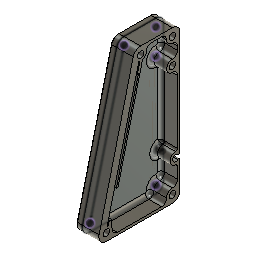
enclosure (Autodesk Fusion 360 design; units mm, degrees)
Autodesk Fusion 360 part; units mm, degrees
sketch "base-measurements" plane through (0, 0, 0) normal (1, 0, 0) x (0, 1, 0)
  circle A0 centre (0, 0) radius 2.55
  circle A1 centre (0, 108) radius 2.55
  circle A2 centre (-25.072576, 108) radius 2.55
  circle A3 centre (-52, 0) radius 2.55
  line L0 (0, 108) -> (-25.072576, 108) construction
  line L1 (-25.072576, 108) -> (-52, 0) construction
  line L2 (-52, 0) -> (0, 0) construction
  circle A4 centre (0, 88) radius 2.55
  line L3 (0, 0) -> (0, 88) construction
  line L4 (0, 88) -> (0, 108) construction
  dimension "rodOuterDiameter" = 5.1
  dimension "d2" = 5.1
  dimension "d3" = 5.1
  dimension "d4" = 5.1
  dimension "d8" = 52
  dimension "d9" = 108
  dimension "d105" = 76
  dimension "d108" = 5.1
  dimension "d134" = 20
  constraint coincident A0.centre L2.end
  constraint coincident A1.centre L0.start
  constraint horizontal L0
  constraint coincident A3.centre L1.end
  constraint horizontal L2
  constraint coincident A4.centre L3.end
  constraint vertical L4
  constraint vertical L3
  measures "rodOuterDiameter" diameter of A0
  measures "d2" diameter of A1
  measures "d3" diameter of A2
  measures "d4" diameter of A3
  measures "d8" distance of A0.centre A3.centre
  measures "d9" distance of A0.centre A1.centre
  measures "d105" angle of L1 L2
  measures "d108" diameter of A4
  measures "d134" distance of A1.centre A4.centre
sketch "left-panel-outline" plane through (0, 0, 0) normal (1, 0, 0) x (0, 1, 0)
  line L0 (-52, -6) -> (0, -6)
  line L1 (0, 114) -> (-25.072576, 114)
  line L2 (-30.89435, 109.451531) -> (-57.821774, 1.451531)
  arc A0 (0, -6) -> (6, 0) centre (0, 0) ccw
  arc A1 (-57.821774, 1.451531) -> (-52, -6) centre (-52, 0) ccw
  arc A2 (6, 108) -> (0, 114) centre (0, 108) ccw
  arc A3 (-25.072576, 114) -> (-30.89435, 109.451531) centre (-25.072576, 108) ccw
  circle A4 centre (0, 108) radius 2.55
  circle A5 centre (-25.072576, 108) radius 2.55
  circle A6 centre (0, 0) radius 2.55
  circle A7 centre (-52, 0) radius 2.55
  circle A8 centre (-25.072576, 108) radius 1.75
  circle A9 centre (0, 108) radius 1.75
  circle A10 centre (0, 0) radius 1.75
  circle A11 centre (-52, 0) radius 1.75
  line L3 (-26.513946, 104.079095) -> (-51.431901, 4.138636)
  line L4 (-26.513946, 104.079095) -> (-25.64068, 103.861366)
  line L5 (-25.640679, 103.861365) -> (-50.558634, 3.920906)
  line L6 (-50.558634, 3.920906) -> (-51.4319, 4.138635)
  line L7 (-25.072578, 108.000001) -> (-26.077313, 103.970231) construction
  line L8 (-52.000001, 0) -> (-50.995267, 4.02977) construction
  circle A12 centre (0, 88) radius 1.75
  circle A13 centre (0, 88) radius 2.55
  line L9 (6, 0) -> (6, 21)
  line L10 (6, 108) -> (6, 26.25)
  arc A14 (4.338562, 25.5) -> (6, 26.25) centre (5, 26.25) ccw
  arc A15 (6, 21) -> (4.338562, 21.75) centre (5, 21) ccw
  arc A16 (4.338562, 25.5) -> (4.338562, 21.75) centre (2.684968, 23.625) ccw
  line L11 (5, 26.25) -> (5, 21) construction
  dimension "d10" = 6
  dimension "screwHole" = 3.5
  dimension "d12" = 3.5
  dimension "d13" = 3.5
  dimension "d14" = 3.5
  dimension "d17" = 103
  dimension "d18" = 0.9
  dimension "d110" = 3.5
  dimension "d122" = 2.5
  dimension "d123" = 1
  dimension "d124" = 21
  dimension "d125" = 5.25
  constraint horizontal L0
  constraint horizontal L1
  constraint tangent L0 A0
  constraint tangent L0 A1
  constraint tangent L1 A2
  constraint tangent L1 A3
  constraint concentric A2 A4
  constraint concentric A3 A5
  constraint concentric A0 A6
  constraint concentric A1 A7
  constraint tangent L2 A1
  constraint tangent L2 A3
  constraint concentric A3 A8
  constraint concentric A4 A9
  constraint concentric A6 A10
  constraint concentric A1 A11
  constraint parallel L3 L5
  constraint perpendicular L5 L6
  constraint perpendicular L3 L4
  constraint coincident A1.centre A7.centre
  constraint equal L7 L8
  constraint parallel L2 L3
  constraint parallel L3 L8
  constraint concentric A12 A13
  constraint tangent A0 L9
  constraint vertical L9
  constraint tangent A2 L10
  constraint vertical L10
  constraint tangent L10 A14
  constraint tangent L9 A15
  constraint tangent A15 A16
  constraint tangent A14 A16
  constraint equal A14 A15
  constraint coincident A14.centre L11.start
  constraint coincident A15.centre L11.end
  constraint vertical L11
  measures "d10" radius of A2
  measures "screwHole" diameter of A8
  measures "d12" diameter of A9
  measures "d13" diameter of A10
  measures "d14" diameter of A11
  measures "d110" diameter of A12
  measures "d122" radius of A16
  measures "d123" radius of A14
  measures "d124" distance of A0.end L9.end
  measures "d125" distance of A14.centre A15.centre
extrude "Extrude1" add sketch "left-panel-outline" against normal blind 5 contours L0 L1 L2 A0 A1 A2 A3 L9 L10 A14 A15 A16 | A4 | A5 | A6 | A7 | L3 L4 L5 L6 | A13 picked at (-17.305036, 38.349698) picked at (-1.246633, 109.90586) picked at (-23.825943, 109.90586) picked at (2.267324, -0.213627) picked at (-49.732676, -0.213627) picked at (-42.543738, 37.306969) picked at (-1.246633, 89.90586) makes body 1
extrude "Extrude2" add sketch "left-panel-outline" along normal blind 13 contours L0 L1 L2 A0 A1 A2 A3 L9 L10 A14 A15 A16 picked at (-17.305036, 38.349698) bodies 1
sketch "left-panel-recess" plane through (13, 0, 0) normal (1, 0, 0) x (0, 1, 0)
  circle A0 centre (-25.072576, 108) radius 2.55
  circle A1 centre (0, 108) radius 2.55
  circle A2 centre (0, 0) radius 2.55
  circle A3 centre (-52, 0) radius 2.55
  line L0 (-51.4319, 4.138635) -> (-26.513946, 104.079095)
  line L1 (-26.513946, 104.079095) -> (-25.640679, 103.861365)
  line L2 (-25.640679, 103.861365) -> (-50.558634, 3.920906)
  line L3 (-50.558634, 3.920906) -> (-51.4319, 4.138635)
  arc A4 (-25.072576, 114) -> (-30.89435, 109.451531) centre (-25.072576, 108) ccw
  line L4 (-30.89435, 109.451531) -> (-57.821774, 1.451531)
  arc A5 (-57.821774, 1.451531) -> (-52, -6) centre (-52, 0) ccw
  line L5 (-52, -6) -> (0, -6)
  arc A6 (0, -6) -> (6, 0) centre (0, 0) ccw
  arc A7 (6, 108) -> (0, 114) centre (0, 108) ccw
  line L6 (0, 114) -> (-25.072576, 114)
  line L7 (-23.747087, 103.189014) -> (-42.942712, 26.199571)
  line L8 (-43.45, -4) -> (-8.55, -4)
  arc A8 (0, 4.55) -> (-4.55, 0) centre (0, 0) ccw
  arc A9 (0, 4.55) -> (4, 8.55) centre (0, 8.55) ccw
  arc A10 (-8.55, -4) -> (-4.55, 0) centre (-8.55, 0) ccw
  arc A11 (-4.55, 108) -> (0, 103.45) centre (0, 108) ccw
  arc A12 (4, 99.45) -> (0, 103.45) centre (0, 99.45) ccw
  line L9 (-16.522576, 112) -> (-8.55, 112)
  arc A13 (-4.55, 108) -> (-8.55, 112) centre (-8.55, 108) ccw
  line L10 (-50.558634, 3.920906) -> (-25.640679, 103.861365)
  arc A14 (-23.190446, 103.857526) -> (-20.522576, 108) centre (-25.072576, 108) ccw
  arc A15 (-16.522576, 112) -> (-20.522576, 108) centre (-16.522576, 108) ccw
  arc A16 (-23.190446, 103.857526) -> (-23.747087, 103.189014) centre (-22.77679, 102.947091) ccw
  arc A17 (-47.45, 0) -> (-47.94694, 2.067657) centre (-52, 0) ccw
  arc A18 (-47.45, 0) -> (-43.45, -4) centre (-43.45, 0) ccw
  line L11 (-48.264993, 4.853065) -> (-47.781149, 6.793656)
  arc A19 (-48.264993, 4.853065) -> (-47.94694, 2.067657) centre (-44.38381, 3.885377) ccw
  line L12 (-44.155581, 26.501973) -> (-26.848332, 95.917558)
  line L13 (-26.848332, 95.917558) -> (-27.576054, 96.099)
  line L14 (-42.942712, 26.199571) -> (-44.155581, 26.501973)
  line L15 (-47.781149, 6.793656) -> (-49.721741, 7.2775)
  line L16 (4, 99.45) -> (4, 96.55)
  arc A20 (4, 79.45) -> (0, 83.45) centre (0, 79.45) ccw
  arc A21 (0, 92.55) -> (4, 96.55) centre (0, 96.55) ccw
  arc A22 (0, 92.55) -> (0, 83.45) centre (0, 88) ccw
  circle A23 centre (0, 88) radius 2.55
  circle A24 centre (0, 88) radius 2.55
  line L17 (6, 0) -> (6, 21)
  arc A25 (6, 21) -> (4.338562, 21.75) centre (5, 21) ccw
  arc A26 (4.338562, 25.5) -> (4.338562, 21.75) centre (2.684968, 23.625) ccw
  arc A27 (4.338562, 25.5) -> (6, 26.25) centre (5, 26.25) ccw
  line L18 (6, 26.25) -> (6, 108)
  arc A28 (2.546242, 28.122861) -> (2.546242, 19.127139) centre (2.684968, 23.625) ccw
  arc A29 (2.546242, 28.122861) -> (4, 29.622148) centre (2.5, 29.622148) ccw
  arc A30 (4, 17.627852) -> (2.546242, 19.127139) centre (2.5, 17.627852) ccw
  line L19 (4, 17.627852) -> (4, 8.55)
  line L20 (4, 29.622148) -> (4, 79.45)
  dimension "d28" = 2
  dimension "d29" = 4
  dimension "d31" = 2
  dimension "d33" = 2
  dimension "d34" = 2
  dimension "d35" = 1
  dimension "d50" = 2
  dimension "d59" = 0.75
  dimension "d60" = 8
  dimension "d71" = 20
  dimension "d112" = 2
  dimension "d117" = 2
  dimension "d118" = 2
  dimension "d119" = 2
  dimension "d126" = 2
  dimension "d127" = 2
  dimension "d128" = 2
  dimension "d129" = 2
  dimension "d130" = 1.5
  constraint horizontal L8
  constraint tangent A8 A9
  constraint tangent A8 A10
  constraint tangent L8 A10
  constraint equal A9 A10
  constraint tangent A11 A12
  constraint equal A9 A12
  constraint horizontal L9
  constraint tangent L9 A13
  constraint equal A12 A13
  constraint tangent A11 A13
  constraint parallel L2 L7
  constraint concentric A0 A14
  constraint tangent A14 A15
  constraint tangent L9 A15
  constraint equal A13 A15
  constraint tangent L7 A16
  constraint tangent A14 A16
  constraint tangent L8 A18
  constraint tangent A17 A18
  constraint equal A10 A18
  constraint tangent L11 A19
  constraint collinear L7 L11
  constraint tangent A17 A19
  constraint equal A18 A19
  constraint perpendicular L2 L13
  constraint perpendicular L12 L13
  constraint perpendicular L12 L14
  constraint perpendicular L2 L15
  constraint tangent A12 L16
  constraint tangent L16 A21
  constraint concentric A22 A23
  constraint coincident A20.end A22.end
  constraint tangent A21 A22
  constraint tangent A20 A22
  constraint equal A12 A21
  constraint equal A20 A21
  constraint tangent A28 A29
  constraint tangent A28 A30
  constraint vertical L19
  constraint tangent A30 L19
  constraint vertical L20
  constraint tangent A29 L20
  constraint coincident A20.start L20.end
  constraint tangent A20 L20
  constraint equal A29 A30
  constraint tangent A9 L19
  measures "d28" distance of L5 L8
  measures "d29" radius of A9
  measures "d31" distance of L6 L9
  measures "d33" distance of L7 L10
  measures "d34" distance of A0 A14
  measures "d35" radius of A16
  measures "d71" distance of L14 L15
  measures "d112" distance of A22 A23
  measures "d117" distance of A1 A11
  measures "d118" distance of A2 A8
  measures "d119" distance of A3 A17
  measures "d126" distance of L16 L18
  measures "d127" distance of L18 L20
  measures "d128" distance of L17 L19
  measures "d129" distance of A26 A28
  measures "d130" radius of A29
extrude "Extrude3" cut sketch "left-panel-recess" against normal blind 13 contours L2 L7 L8 A8 A9 A10 A11 A12 L9 A13 L10 A14 A15 A16 A17 A18 L11 A19 L12 L13 L14 L15 L16 A20 A21 A22 A28 A29 A30 L19 L20 picked at (-15.142097, 45.9114) bodies 1
ref_plane "WorkPlane1" through (151, -23.715951, 54) normal (1, 0, 0) x (0, 1, 0)
sketch "right-panel" plane through (151, 0, 0) normal (1, 0, 0) x (0, 1, 0)
  arc A0 (6, 108) -> (0, 114) centre (0, 108) ccw
  line L0 (0, 114) -> (-25.072576, 114)
  arc A1 (-25.072576, 114) -> (-30.89435, 109.451531) centre (-25.072576, 108) ccw
  line L1 (-30.89435, 109.451531) -> (-57.821774, 1.451531)
  arc A2 (-57.821774, 1.451531) -> (-52, -6) centre (-52, 0) ccw
  line L2 (-52, -6) -> (0, -6)
  arc A3 (0, -6) -> (6, 0) centre (0, 0) ccw
  circle A4 centre (-25.072576, 108) radius 2.55
  circle A5 centre (-25.072576, 108) radius 1.75
  circle A6 centre (0, 108) radius 2.55
  circle A7 centre (0, 108) radius 1.75
  line L3 (-26.513946, 104.079095) -> (-51.431901, 4.138636)
  line L4 (-26.513946, 104.079095) -> (-25.64068, 103.861366)
  line L5 (-50.558634, 3.920906) -> (-51.4319, 4.138635)
  line L6 (-25.640679, 103.861365) -> (-50.558634, 3.920906)
  circle A8 centre (0, 0) radius 2.55
  circle A9 centre (0, 0) radius 1.75
  circle A10 centre (-52, 0) radius 2.55
  circle A11 centre (-52, 0) radius 1.75
  line L7 (-52, 0) -> (-50.995267, 4.02977)
  line L8 (-25.072578, 108.000001) -> (-26.077313, 103.970231)
  circle A12 centre (0, 88) radius 2.55
  circle A13 centre (0, 88) radius 1.75
  line L9 (6, 108) -> (6, 0)
  constraint coincident A0.start L9.start
  constraint coincident A3.end L9.end
extrude "Extrude6" add sketch "right-panel" along normal blind 5 separate body contours A0 L0 A1 L1 A2 L2 A3 L9 | A4 | A6 | L3 L4 L5 L6 | A8 | A10 | A12 picked at (-17.702878, 30.640302) picked at (-25.745071, 105.824135) picked at (-1.246633, 109.90586) picked at (-42.834827, 37.379546) picked at (2.267324, -0.213627) picked at (-50.655141, 1.838083) picked at (-1.246633, 89.90586) makes body 2
extrude "Extrude7" add sketch "right-panel" against normal blind 13 separate body contours A0 L0 A1 L1 A2 L2 A3 L9 picked at (-17.702878, 30.640302) makes body 3
extrude "Extrude8" add sketch "right-panel" against normal blind 9.5 contours L3 L4 L5 L6 picked at (-42.834827, 37.379546) bodies 2 3
sketch "right-panel-recess" plane through (138, 0, 0) normal (-1, 0, 0) x (0, -1, 0)
  circle A0 centre (25.072576, 108) radius 2.55
  circle A1 centre (0, 0) radius 2.55
  line L0 (26.513946, 104.079095) -> (51.4319, 4.138635)
  line L1 (51.4319, 4.138635) -> (50.558634, 3.920906)
  line L2 (50.558634, 3.920906) -> (25.640679, 103.861365)
  line L3 (25.640679, 103.861365) -> (26.513946, 104.079095)
  circle A2 centre (52, 0) radius 2.55
  circle A3 centre (0, 108) radius 2.55
  arc A4 (-6, 0) -> (0, -6) centre (0, 0) ccw
  line L4 (0, -6) -> (52, -6)
  arc A5 (52, -6) -> (57.821774, 1.451531) centre (52, 0) ccw
  line L5 (57.821774, 1.451531) -> (30.89435, 109.451531)
  arc A6 (30.89435, 109.451531) -> (25.072576, 114) centre (25.072576, 108) ccw
  line L6 (25.072576, 114) -> (0, 114)
  arc A7 (0, 114) -> (-6, 108) centre (0, 108) ccw
  arc A8 (47.94694, 2.067657) -> (47.45, 0) centre (52, 0) ccw
  arc A9 (43.45, -4) -> (47.45, 0) centre (43.45, 0) ccw
  line L7 (43.45, -4) -> (8.55, -4)
  arc A10 (4.55, 0) -> (8.55, -4) centre (8.55, 0) ccw
  arc A11 (4.55, 0) -> (0, 4.55) centre (0, 0) ccw
  arc A12 (-4, 8.55) -> (0, 4.55) centre (0, 8.55) ccw
  arc A13 (0, 103.45) -> (-4, 99.45) centre (0, 99.45) ccw
  arc A14 (0, 103.45) -> (4.55, 108) centre (0, 108) ccw
  arc A15 (8.55, 112) -> (4.55, 108) centre (8.55, 108) ccw
  line L8 (16.522576, 112) -> (8.55, 112)
  arc A16 (20.522576, 108) -> (16.522576, 112) centre (16.522576, 108) ccw
  line L9 (23.858089, 102.743812) -> (48.264993, 4.853065)
  arc A17 (20.522576, 108) -> (22.880881, 104.012648) centre (25.072576, 108) ccw
  arc A18 (23.858089, 102.743812) -> (22.880881, 104.012648) centre (21.9175, 102.259969) ccw
  arc A19 (47.94694, 2.067657) -> (48.264993, 4.853065) centre (44.38381, 3.885377) ccw
  arc A20 (0, 83.45) -> (-4, 79.45) centre (0, 79.45) ccw
  arc A21 (0, 83.45) -> (0, 92.55) centre (0, 88) ccw
  arc A22 (-4, 96.55) -> (0, 92.55) centre (0, 96.55) ccw
  line L10 (-4, 99.45) -> (-4, 96.55)
  circle A23 centre (0, 88) radius 2.55
  circle A24 centre (0, 88) radius 2.55
  line L11 (-6, 108) -> (-6, 0)
  line L12 (-4, 79.45) -> (-4, 8.55)
  point P0 (0, 88)
  dimension "d67" = 2
  dimension "d68" = 2
  constraint parallel L2 L9
  constraint concentric A0 A17
  constraint tangent A17 A18
  constraint tangent L9 A18
  constraint tangent L9 A19
  constraint tangent A8 A19
  constraint coincident A20.end L12.start
  constraint coincident A12.start L12.end
  measures "d67" distance of L2 L9
  measures "d68" radius of A18
extrude "Extrude9" cut sketch "right-panel-recess" against normal blind 13.5 contours A8 A9 L7 A10 A11 A12 A13 A14 A15 L8 A16 L9 A17 A18 A19 A20 A21 A22 L10 L12 picked at (13.421664, 30.951022) bodies 2
fillet "Fillet1" radius 3 25 edges at (0, -33.3449, 64.694292) (0, -23.545268, 103.58697) (0, -21.247253, 105.536384) (0, -19.351003, 110.828427) (0, -12.536288, 112) (0, -5.721573, 110.828427) (0, -3.217336, 104.782664) (0, 2.828427, 102.278427) (0, 4, 98) (0, 2.828427, 93.721573) (0, -4.55, 88) (0, 2.828427, 82.278427) (0, 4, 54.536074) (0, 3.576885, 28.577965) (0, -1.815032, 23.625) (0, 3.576885, 18.672035) (0, 4, 13.088926) (0, 2.828427, 5.721573) (0, -3.217336, 3.217336) (0, -5.721573, -2.828427) (0, -26, -4) (0, -46.278427, -2.828427) (0, -47.575979, 1.063268) (0, -48.357986, 3.431584) (0, -48.023071, 5.82336) on bodies 1
fillet "Fillet2" radius 3 20 edges at (151.5, -3.217336, 104.782664) (151.5, -5.721573, 110.828427) (151.5, -12.536288, 112) (151.5, -19.351003, 110.828427) (151.5, -21.156282, 105.683722) (151.5, -23.502034, 103.480314) (151.5, -36.061541, 53.798438) (151.5, -48.357986, 3.431584) (151.5, -47.575979, 1.063268) (151.5, -46.278427, -2.828427) (151.5, -26, -4) (151.5, -5.721573, -2.828427) (151.5, -3.217336, 3.217336) (151.5, 2.828427, 5.721573) (151.5, 4, 44) (151.5, 2.828427, 82.278427) (151.5, -4.55, 88) (151.5, 2.828427, 93.721573) (151.5, 4, 98) (151.5, 2.828427, 102.278427) on bodies 2
sketch "rpi-support-bar" plane through (0, 0, 0) normal (1, 0, 0) x (0, 1, 0)
  arc A0 (6, 88) -> (-1.764706, 82.265385) centre (0, 88) ccw
  line L0 (0, 79.875962) -> (0, 8.124038)
  arc A1 (0, 79.875962) -> (-1.764706, 82.265385) centre (-2.5, 79.875962) ccw
  circle A2 centre (0, 0) radius 2.55 construction
  arc A3 (-1.764706, 5.734615) -> (6, -0.000003) centre (0, 0) ccw
  arc A4 (-1.764706, 5.734615) -> (0, 8.124038) centre (-2.5, 8.124038) ccw
  line L1 (0, 0) -> (0, -6) construction
  circle A5 centre (0, 88) radius 2.55
  circle A6 centre (0, 0) radius 2.55
  circle A7 centre (0, 88) radius 2.55
  line L2 (6, -0.000003) -> (6, 88)
  arc A8 (0, -6) -> (6, 0) centre (0, 0) ccw
  dimension "d100" = 2.5
  dimension "d133" = 6
  constraint vertical L0
  constraint tangent L0 A1
  constraint coincident A2.centre A3.centre
  constraint tangent L0 A4
  constraint coincident A3 L1.end
  constraint vertical L1
  constraint tangent A0 A1
  constraint tangent A3 A4
  constraint equal A1 A4
  constraint concentric A3 A6
  constraint equal A2 A6
  constraint concentric A0 A5
  constraint equal A5 A7
  constraint concentric A5 A7
  constraint equal A0 A3
  constraint tangent A0 L2
  constraint tangent L2 A8
  constraint vertical L2
  constraint coincident A0.start L2.end
  measures "d100" radius of A1
  measures "d133" distance of L0 L2
extrude "Extrude14" add sketch "left-panel-outline" along normal blind 0.5 contours L3 L4 L5 L6 picked at (-42.543738, 37.306969) bodies 1
chamfer "Chamfer11" distance 1.6 distance2 1.6 10 edges at (-5, -1.631573, 107.367173) (-5, -26.704149, 107.367173) (-5, -1.631573, 87.367173) (-5, -1.631573, -0.632827) (-5, -53.631573, -0.632827) (156, -53.631573, 0.632827) (156, -1.631573, 0.632827) (156, -1.631573, 88.632827) (156, -1.631573, 108.632827) (156, -26.704149, 108.632827) measured on face at (-5, -17.501371, 37.822398) measured on face at (-5, -17.501371, 37.822398) measured on face at (-5, -17.501371, 37.822398) measured on face at (-5, -17.501371, 37.822398) measured on face at (-5, -17.501371, 37.822398) measured on face at (156, -17.688826, 29.845799) measured on face at (156, -17.688826, 29.845799) measured on face at (156, -17.688826, 29.845799) measured on face at (156, -17.688826, 29.845799) measured on face at (156, -17.688826, 29.845799) tangent chain off on bodies 1 2
chamfer "Chamfer12" distance 1 distance2 1 20 edges at (-5, 6, 10.5) (-5, 4.242641, -4.242641) (-5, -26, -6) (-5, -56.728065, -3.693969) (-5, -44.358062, 55.451531) (-5, -28.766545, 112.728065) (-5, -12.536288, 114) (-5, 4.242641, 112.242641) (-5, 6, 67.125) (-5, 5.411438, 25.338562) (-5, 0.184968, 23.625) (-5, 5.411438, 21.911438) (156, -26, -6) (156, 4.242641, -4.242641) (156, 6, 54) (156, 4.242641, 112.242641) (156, -12.536288, 114) (156, -28.766545, 112.728065) (156, -44.358062, 55.451531) (156, -56.728064, -3.693969) measured on face at (-5, -17.73249, 37.950019) measured on face at (-5, -17.73249, 37.950019) measured on face at (-5, -17.73249, 37.950019) measured on face at (-5, -17.73249, 37.950019) measured on face at (-5, -17.73249, 37.950019) measured on face at (-5, -17.73249, 37.950019) measured on face at (-5, -17.73249, 37.950019) measured on face at (-5, -17.73249, 37.950019) measured on face at (-5, -17.73249, 37.950019) measured on face at (-5, -17.73249, 37.950019) measured on face at (-5, -17.73249, 37.950019) measured on face at (-5, -17.73249, 37.950019) measured on face at (156, -17.891667, 30.300395) measured on face at (156, -17.891667, 30.300395) measured on face at (156, -17.891667, 30.300395) measured on face at (156, -17.891667, 30.300395) measured on face at (156, -17.891667, 30.300395) measured on face at (156, -17.891667, 30.300395) measured on face at (156, -17.891667, 30.300395) measured on face at (156, -17.891667, 30.300395) tangent chain off on bodies 1 2
extrude "Extrude15" add sketch "rpi-support-bar" along normal blind 6 separate body contours A0 L0 A1 A3 A4 L2 A8 picked at (4, 32.041345) makes body 4
sketch "rpi-holes" plane through (0, 0, 0) normal (0, -1, 0) x (1, 0, 0)
  line L0 (0, 61.875962) -> (0, 8.124038)
  line L1 (0, 8.124038) -> (6, 8.124038)
  line L2 (6, 8.124038) -> (6, 61.875962)
  circle A0 centre (3, 71.875962) radius 3
  line L3 (0, 108) -> (0, 0) construction
  circle A1 centre (3, 71.875962) radius 1.2
  circle A2 centre (3, 48.875962) radius 3
  circle A3 centre (3, 48.875962) radius 1.2
  line L4 (0, 79.875962) -> (0, 8.124038)
  line L5 (0, 8.124038) -> (6, 8.124038)
  line L6 (6, 8.124038) -> (6, 79.875962)
  line L7 (6, 79.875962) -> (0, 79.875962)
  dimension "d89" = 2.4
  dimension "d91" = 2.4
  dimension "d92" = 23
  dimension "d137" = 8
  constraint tangent L2 A0
  constraint tangent A0 L3
  constraint concentric A0 A1
  constraint concentric A2 A3
  constraint tangent L2 A2
  constraint tangent L3 A2
  measures "d89" diameter of A1
  measures "d91" diameter of A3
sketch "rpi-support-bar-usb" plane through (0, 0, 0) normal (1, 0, 0) x (0, 1, 0)
  line L0 (6, -0.000003) -> (6, 88)
  arc A0 (6, 88) -> (-1.764706, 82.265385) centre (0, 88) ccw
  circle A1 centre (0, 88) radius 2.55
  arc A2 (0, 79.875962) -> (-1.764706, 82.265385) centre (-2.5, 79.875962) ccw
  circle A3 centre (0, 0) radius 2.55
  line L1 (0, 79.875962) -> (0, 45.745967)
  arc A4 (-6, 0) -> (6, -0.000003) centre (0, 0) ccw
  line L2 (-6, 0) -> (-6, 38)
  arc A5 (-1.5, 43.809475) -> (-6, 38) centre (0, 38) ccw
  arc A6 (-1.5, 43.809475) -> (0, 45.745967) centre (-2, 45.745967) ccw
  line L3 (5, 5) -> (-5, 5) construction
  line L4 (-5, 5) -> (-5, 43) construction
  line L5 (-5, 43) -> (5, 43) construction
  line L6 (5, 43) -> (5, 5) construction
  circle A7 centre (0, 38) radius 5 construction
  circle A8 centre (0, 38) radius 1.75
  line L7 (-3.5, 17.5) -> (-3.5, 30.5)
  line L8 (-3.5, 30.5) -> (3.5, 30.5)
  line L9 (3.5, 17.5) -> (-3.5, 17.5)
  line L10 (3.5, 30.5) -> (3.5, 17.5)
  line L11 (3.5, 24) -> (5, 24) construction
  line L12 (-3.5, 24) -> (-5, 24) construction
  circle A9 centre (0, 10) radius 5 construction
  circle A10 centre (0, 10) radius 1.75
  dimension "d143" = 10
  dimension "d144" = 38
  dimension "d145" = 3.5
  dimension "d146" = 13
  dimension "d147" = 7
  dimension "d148" = 10
  dimension "d149" = 2
  constraint tangent A2 L1
  constraint coincident A3.centre A4.centre
  constraint tangent L2 A5
  constraint tangent A5 A6
  constraint tangent L1 A6
  constraint equal A4 A5
  constraint tangent A4 L2
  constraint horizontal L5
  constraint vertical L6
  constraint horizontal L3
  constraint vertical L4
  constraint tangent L4 A9
  constraint tangent L4 A7
  constraint tangent L5 A7
  constraint tangent L6 A7
  constraint tangent L6 A9
  constraint tangent L3 A9
  constraint concentric A9 A10
  constraint concentric A7 A8
  constraint equal A8 A10
  constraint horizontal L8
  constraint vertical L10
  constraint horizontal L9
  constraint vertical L7
  constraint midpoint L11.start L10
  constraint midpoint L11.end L6
  constraint horizontal L11
  constraint coincident L12.start L7
  constraint coincident L12.end L4
  constraint perpendicular L4 L12
  constraint midpoint L12.end L4
  constraint equal L11 L12
  constraint concentric A5 A7
  constraint vertical L2
  measures "d143" distance of L4.end L5.end
  measures "d144" distance of L4.end L3.end
  measures "d145" diameter of A10
  measures "d146" distance of L8.end L9.start
  measures "d147" distance of L9.start L7.start
  measures "d148" vertical distance of A3.centre A9.centre
  measures "d149" radius of A6
extrude "Extrude16" add sketch "rpi-support-bar-usb" along normal blind 6 separate body contours L0 A0 A2 L1 A4 L2 A5 A6 picked at (2, 71.207309) makes body 5
extrude "Extrude17" add sketch "rpi-holes" along normal blind 1.5 contours A2 | A0 | A1 | A3 picked at (5.388831, 48.726919) picked at (0.942297, 73.098493) picked at (2.269504, 71.650634) picked at (2.461596, 48.702408) bodies 5
extrude "Extrude18" cut sketch "rpi-holes" along normal blind -5 and the other way blind -3 contours A1 | A3 picked at (2.269504, 71.650634) picked at (2.461596, 48.702408) bodies 5
chamfer "Chamfer13" distance 1 distance2 1 2 edges at (0.203018, -1.5, 47.791115) (0.203018, -1.5, 70.791115) measured on face at (5.388831, -1.5, 49.025004) measured on face at (5.216929, -1.5, 72.778154) tangent chain off on bodies 5
chamfer "Chamfer14" distance 0.5 angle 45 4 edges at (3, 0, 74.875962) (3, 0, 68.875962) (3, 0, 51.875962) (3, 0, 45.875962) tangent chain off on bodies 5
chamfer "Chamfer15" distance 1.6 angle 45 2 edges at (0, -1.631573, 38.632827) (0, -1.631573, 10.632827) tangent chain off on bodies 5
chamfer "Chamfer16" distance 1.6 angle 45 4 edges at (0, 0, 30.5) (0, 3.5, 24) (0, 0, 17.5) (0, -3.5, 24) tangent chain off on bodies 5
extrude "Extrude19" add sketch "rpi-holes" along normal blind 1.5 contours A2 | A0 picked at (5.388831, 48.726919) picked at (0.942297, 73.098493) bodies 4
extrude "Extrude20" cut sketch "rpi-holes" against normal blind 5 contours A1 | A3 picked at (2.269504, 71.650634) picked at (2.461596, 48.702408) bodies 4
chamfer "Chamfer17" distance 1 angle 45 2 edges at (0.203018, -1.5, 70.791115) (0.203018, -1.5, 47.791115) tangent chain off on bodies 4
chamfer "Chamfer18" distance 0.5 angle 45 4 edges at (3, 0, 74.875962) (3, 0, 68.875962) (3, 0, 51.875962) (3, 0, 45.875962) tangent chain off on bodies 4
hidden bodies 2 4 5
equation "d2 = rodOuterDiameter"
equation "d3 = rodOuterDiameter"
equation "d4 = rodOuterDiameter"
equation "d12 = screwHole"
equation "d13 = screwHole"
equation "d14 = screwHole"
equation "sidePanelThickness = -5 mm"
equation "screwRecess = 1.6 mm"
equation "innerRecessDistance = 2 mm"
equation "d28 = innerRecessDistance"
equation "d31 = innerRecessDistance"
equation "d33 = innerRecessDistance"
equation "d34 = innerRecessDistance"
equation "leftPanelRecess = -13 mm"
equation "d56 = -sidePanelThickness"
equation "d67 = innerRecessDistance"
equation "innerRecessFillet = 3 mm"
equation "d75 = innerRecessFillet"
equation "d108 = rodOuterDiameter"
equation "d110 = screwHole"
equation "d112 = innerRecessDistance"
equation "d117 = innerRecessDistance"
equation "d118 = innerRecessDistance"
equation "d119 = innerRecessDistance"
equation "d120 = screwRecess"
equation "d126 = innerRecessDistance"
equation "d127 = innerRecessDistance"
equation "d128 = innerRecessDistance"
equation "d129 = innerRecessDistance"
equation "d161 = screwRecess"
named bodies: "left-panel", "right-panel", "rpi-support-bar", "rpi-support-bar-usb"
